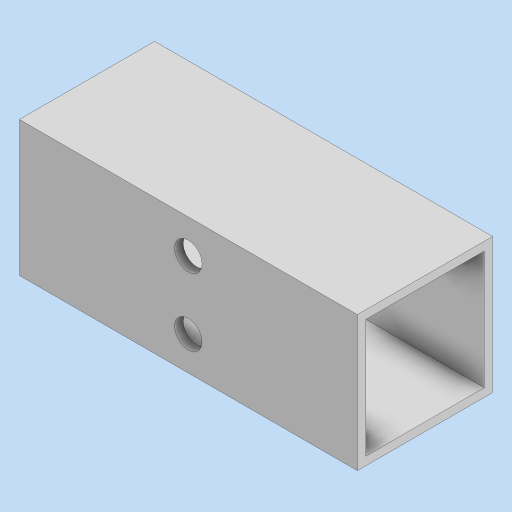
# Autodesk Inventor part: 1inTubeBase
Saved by Autodesk Inventor 2024 (Build 280153000, 153)
## iProperties
Created: 2024-01-10
Part Number: 1inTubeBase
Material: Generic
Document SubType Name: Modeling
Designer: megan
Density: 1 g/cm^3
Appearance: Default
Author: megan
Autodesk Inventor part; units mm, degrees
ref_plane "YZ Plane" through (0, 0, 0) normal (1, 0, 0) x (0, 1, 0)
ref_plane "XZ Plane" through (0, 0, 0) normal (0, 1, 0) x (-1, 0, 0)
ref_plane "XY Plane" through (0, 0, 0) normal (0, 0, 1) x (1, 0, 0)
sketch "Sketch1" plane through (0, 0, 0) normal (1, 0, 0) x (0, 1, 0)
  line L0 (0, 0) -> (25.4, 0)
  line L1 (25.4, 0) -> (25.4, -25.4)
  line L2 (25.4, -25.4) -> (0, -25.4)
  line L3 (0, -25.4) -> (0, 0)
  line L4 (23.8125, -23.8125) -> (23.8125, -1.5875)
  line L5 (23.8125, -1.5875) -> (1.5875, -1.5875)
  line L6 (1.5875, -1.5875) -> (1.5875, -23.8125)
  line L7 (1.5875, -23.8125) -> (23.8125, -23.8125)
  dimension "d0" = 25.4
  dimension "d1" = 25.4
  dimension "d2" = 1.5875
  constraints: 16 end point, 4 parallel, 2 perpendicular, 1 horizontal, 3 other
  measures "d0" distance of L1.end L2.end
  measures "d1" distance of L0.end L1.end
  measures "d2" distance between parallel lines of L1 L4
extrude "Extrusion1" add sketch "Sketch1" along normal mid plane 63.5
sketch "Sketch2" plane through (-31.75, 0, 0) normal (0, 0, 1) x (1, 0, 0)
  circle A0 centre (31.75, 6.35) radius 2.5781
  circle A1 centre (31.75, 19.05) radius 2.5781
  line L0 (0, 25.4) -> (63.5, 25.4) projected
  line L1 (0, 0) -> (63.5, 0) projected
  line L2 (63.5, 25.4) -> (63.5, 0) projected
  point P0 (31.75, 0)
  dimension "d6" = 5.1562
  dimension "d7" = 5.1562
  dimension "d8" = 6.35
  dimension "d9" = 6.35
  dimension "d10" = 31.75
  dimension "d11" = 31.75
  constraints: 2 centre point
  measures "d6" diameter of A0
  measures "d7" diameter of A1
  measures "d8" distance from line of L0 A1.centre
  measures "d9" distance from line of L1 A0.centre
  measures "d10" distance from line of L2 A0.centre
  measures "d11" distance from line of L2 A1.centre
extrude "Extrusion2" cut sketch "Sketch2" against normal through all
equation "\"d11\" = d10"
body "Solid1"
